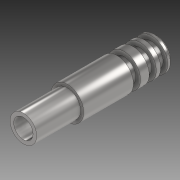
# Autodesk Inventor part: 11310_Pipe Inserts_V1
Saved by Autodesk Inventor 2020 (Build 240168000, 168)
## iProperties
Created: 2019-06-06
Part Number: 11310_Pipe Inserts_V1
Material: Stainless Steel, Austenitic
Document SubType Name: Modeling
Designer: e22ma
Density: 8 g/cm^3
Appearance: Semi-Polished
Author: e22ma
Autodesk Inventor part; units mm, degrees
ref_plane "YZ Plane" through (0, 0, 0) normal (1, 0, 0) x (0, 1, 0)
ref_plane "XZ Plane" through (0, 0, 0) normal (0, 1, 0) x (-1, 0, 0)
ref_plane "XY Plane" through (0, 0, 0) normal (0, 0, 1) x (1, 0, 0)
sketch "Sketch1" plane through (0, 0, 0) normal (1, 0, 0) x (0, 1, 0)
  line L0 (-2.3153, 0) -> (7.2097, 0) projected
  line L1 (7.2097, -18.2) -> (-2.3153, -18.2) projected
  line L2 (2.4472, 0) -> (2.4472, -25.82)
  line L3 (-0.3468, 0) -> (-0.3468, -25.82)
  line L4 (-0.3468, -25.82) -> (-2.2772, -25.82)
  line L5 (-2.2772, -25.82) -> (-2.2772, 0)
  line L6 (-2.2772, 0) -> (-0.3468, 0)
  line L7 (-2.2772, -24.296) -> (-0.9818, -24.296)
  line L8 (-0.9818, -24.296) -> (-0.9818, -22.264)
  line L9 (-0.9818, -22.264) -> (-2.2772, -22.264)
  line L10 (-2.2772, -22.264) -> (-2.2772, -24.296)
  line L11 (-2.2772, -20.994) -> (-0.9818, -20.994)
  line L12 (-0.9818, -20.994) -> (-0.9818, -18.962)
  line L13 (-0.9818, -18.962) -> (-2.2772, -18.962)
  line L14 (-2.2772, -18.962) -> (-2.2772, -20.994)
  line L15 (-2.2772, -16.422) -> (-0.9818, -16.422)
  line L16 (-0.9818, -16.422) -> (-0.9818, -14.39)
  line L17 (-0.9818, -14.39) -> (-2.2772, -14.39)
  line L18 (-2.2772, -14.39) -> (-2.2772, -16.422)
  point P0 (0, 0)
  dimension "d0" = 7.62
  dimension "d1" = 5.588
  dimension "d2" = 9.4488
  dimension "d3" = 2.032
  dimension "d4" = 1.27
  dimension "d5" = 2.032
  dimension "d6" = 0.635
  dimension "d7" = 1.524
  dimension "d8" = 2.54
  dimension "d9" = 2.032
  constraints: 34 end point, 7 parallel, 6 point on line, 4 horizontal, 4 perpendicular, 3 vertical, 1 collinear, 1 midpoint
  measures "d0" distance from line of L2.end L1
  measures "d1" diameter of L3 L2
  measures "d2" diameter of L4.end L2
  measures "d3" distance of L8.end L7.end
  measures "d4" distance between parallel lines of L9 L11
  measures "d5" distance of L11.end L12.end
  measures "d6" distance between parallel lines of L3 L8
  measures "d7" distance between parallel lines of L4 L7
  measures "d8" distance between parallel lines of L13 L15
  measures "d9" distance of L15.end L16.end
revolve "Revolution1" add sketch "Sketch1" angle 360 about axis through (0, 2.4472, 0) along (0, 0, -1) contours L0 L3 L1 L5 L15 L16 L17 | L3 L4 L5 L7 L8 L9 L11 L12 L13 L1
chamfer "Chamfer1" distance 0.762 angle 45 1 edges at (0, 7.1716, -25.82)
sketch "Sketch5" plane through (0, 2.4472, 0) normal (0, 0, 1) x (1, 0, 0)
  circle A0 centre (0, 0) radius 4.7244 projected
  circle A1 centre (0, 0) radius 2.794 projected
  circle A2 centre (0, 0) radius 3.8545
  point P0 (0, -2.4472)
  dimension "d22" = 0.87
  constraints: 1 centre point
  measures "d22" radial gap between concentric circles of A0 A2
extrude "Extrusion2" add sketch "Sketch5" along normal blind 12.7 contours A2
equation "\"d5\" = d3"
equation "\"d9\" = d3"
body "Solid1"
